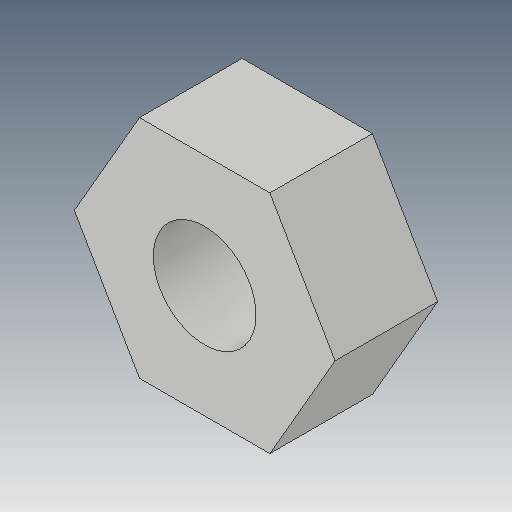
# Autodesk Inventor part: m3 nut
Saved by Autodesk Inventor 2020.3 (Build 243373000, 373)
## iProperties
Created: 2021-02-26
Part Number: m3 nut
Material: Generic
Document SubType Name: Modeling
Designer: paulg
Density: 1 g/cm^3
Appearance: Default
Author: paulg
Autodesk Inventor part; units mm, degrees
ref_plane "YZ Plane" through (0, 0, 0) normal (1, 0, 0) x (0, 1, 0)
ref_plane "XZ Plane" through (0, 0, 0) normal (0, 1, 0) x (-1, 0, 0)
ref_plane "XY Plane" through (0, 0, 0) normal (0, 0, 1) x (1, 0, 0)
sketch "Sketch1" plane through (0, 0, 0) normal (0, 0, 1) x (1, 0, 0)
  line L0 (-1.5877, 2.75) -> (1.5877, 2.75)
  line L1 (1.5877, 2.75) -> (3.1754, 0)
  line L2 (3.1754, 0) -> (1.5877, -2.75)
  line L3 (1.5877, -2.75) -> (-1.5877, -2.75)
  line L4 (-1.5877, -2.75) -> (-3.1754, 0)
  line L5 (-3.1754, 0) -> (-1.5877, 2.75)
  circle A0 centre (0, 0) radius 1.25
  dimension "d0" = 5.5
  dimension "d1" = 2.5
  constraints: 12 end point, 2 coincident, 1 centre point, 1 horizontal, 13 other
  measures "d0" distance between parallel lines of L3 L0
  measures "d1" diameter of A0
extrude "Extrusion1" add sketch "Sketch1" along normal blind 2.5
body "Solid1"
